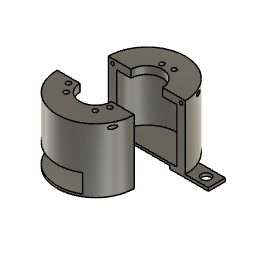
RotaryEncoderHolderCombined (Autodesk Fusion 360 design; units mm, degrees)
Autodesk Fusion 360 part; units mm, degrees
note: some values were not read from the file. Set by a fixed rule: which sketch regions a step uses.
sketch "Sketch1" plane through (0, 0, 0) normal (0, 0, 1) x (1, 0, 0)
  arc A0 (-25, 0) -> (25, 0) centre (0, 0) ccw
  line L0 (-25, 0) -> (25, 0)
  dimension "d3" = 50
  constraint coincident A0.centre origin
  constraint horizontal L0
  measures "d3" distance of A0.start A0.end
extrude "Extrude1" add sketch "Sketch1" along normal blind 41.5 makes body 1
sketch "Sketch2" plane through (0, 0, 41.5) normal (0, 0, 1) x (-1, 0, 0)
  arc A0 (25, 0) -> (-25, 0) centre (0, 0) ccw
  line L0 (-25, 0) -> (25, 0)
  circle A1 centre (0, 0) radius 19.5
  dimension "d6" = 39
  constraint coincident A0.centre A1.centre
  measures "d6" diameter of A1
extrude "Extrude2" cut sketch "Sketch2" against normal blind 35 from surface at -5 contours L0 A1 picked at (5.8563, 2.8202) bodies 1
sketch "Sketch5" plane through (0, 0, 41.5) normal (0, 0, 1) x (-1, 0, 0)
  arc A0 (25, 0) -> (-25, 0) centre (0, 0) ccw
  line L0 (-25, 0) -> (25, 0)
  circle A1 centre (0, 0) radius 10.25
  dimension "d10" = 20.5
  constraint coincident A0.centre A1.centre
  measures "d10" diameter of A1
extrude "Extrude3" cut sketch "Sketch5" against normal blind 5 contours L0 A1 picked at (0.2553, 3.4071) bodies 1
ref_plane "WorkPlane1" through (0, 0, 0) normal (0, 1, 0) x (0, 0, 1)
sketch "Sketch8" plane through (0, 0, 0) normal (0, 1, 0) x (-1, 0, 0)
  line L0 (-10.25, 36.5) -> (-10.25, 41.5)
  line L1 (-10.25, 41.5) -> (-25, 41.5)
  line L2 (-25, 41.5) -> (-25, 0)
  line L3 (-25, 0) -> (25, 0)
  line L4 (25, 0) -> (25, 41.5)
  line L5 (25, 41.5) -> (10.25, 41.5)
  line L6 (10.25, 41.5) -> (10.25, 36.5)
  line L7 (10.25, 36.5) -> (19.5, 36.5)
  line L8 (19.5, 36.5) -> (19.5, 1.5)
  line L9 (19.5, 1.5) -> (-19.5, 1.5)
  line L10 (-19.5, 1.5) -> (-19.5, 36.5)
  line L11 (-19.5, 36.5) -> (-10.25, 36.5)
  circle A0 centre (22.25, 38.75) radius 1.1
  line L12 (0, 46.5) -> (0, -12.5) construction
  line L13 (-30, 19) -> (33, 19) construction
  circle A1 centre (-22.25, 38.75) radius 1.1
  dimension "d40" = 2.2
  dimension "d41" = 2.75
  dimension "d42" = 2.75
  dimension "d43" = 22.5
  dimension "d44" = 22.25
  constraint perpendicular L3 L12
  constraint horizontal L13
  constraint symmetric A0 L12 A1
  measures "d40" diameter of A0
  measures "d41" distance of L4 A0.centre
  measures "d42" distance of L5 A0.centre
  measures "d43" distance of L1 L13
  measures "d44" distance of A0.centre L12
extrude "Extrude5" cut sketch "Sketch8" against normal blind 14 contours A0 | A1 bodies 1
mirror "Mirror1" about plane through (0, 0, 0) normal (0, 1, 0) of bodies 1 makes body 2
sketch "Sketch6" plane through (0, 0, 41.5) normal (0, 0, 1) x (-1, 0, 0)
  arc A0 (10.25, 0) -> (-10.25, 0) centre (0, 0) ccw
  line L0 (10.25, 0) -> (25, 0)
  arc A1 (25, 0) -> (-25, 0) centre (0, 0) ccw
  line L1 (-25, 0) -> (-10.25, 0)
  circle A2 centre (-12.968, 3.7525) radius 1.5
  circle A3 centre (-10.1336, 10.3711) radius 1.5
  circle A4 centre (14.0483, 3.5909) radius 1.5
  circle A5 centre (9.7334, 9.3547) radius 1.5
  dimension "d16" = 13.5
  dimension "d17" = 14.5
  dimension "d18" = 3
  dimension "d19" = 3
  dimension "d20" = 7.2
  dimension "d22" = 3
  dimension "d23" = 3
  dimension "d24" = 14.5
  dimension "d25" = 13.5
  dimension "d26" = 7.2
  dimension "d28" = 19.893
  dimension "d37" = 3.7525
  measures "d16" distance of A0.centre A2.centre
  measures "d17" distance of A0.centre A3.centre
  measures "d18" diameter of A2
  measures "d19" diameter of A3
  measures "d20" distance of A2.centre A3.centre
  measures "d22" diameter of A4
  measures "d23" diameter of A5
  measures "d24" distance of A0.centre A4.centre
  measures "d25" distance of A0.centre A5.centre
  measures "d26" distance of A4.centre A5.centre
  measures "d28" distance of A3.centre A5.centre
  measures "d37" distance of L1 A2.centre
ref_plane "WorkPlane2" through (0, -12.5, 41.5) normal (0, 0, 1) x (-1, 0, 0)
sketch "Sketch7" plane through (0, -11.5, 41.5) normal (0, 0, 1) x (1, 0, 0)
  circle A0 centre (-3.2352, 24.6066) radius 1.5
  circle A1 centre (3.9139, 25.4618) radius 1.5
  point P0 (0, 11.5)
  point P1 (-14.0483, 7.9091)
  dimension "d30" = 3
  dimension "d31" = 3
  dimension "d32" = 13.5
  dimension "d33" = 14.5
  dimension "d35" = 7.2
  dimension "d36" = 19.893
  measures "d30" diameter of A0
  measures "d31" diameter of A1
  measures "d32" distance of A0.centre P0
  measures "d33" distance of A1.centre P0
  measures "d35" distance of A0.centre A1.centre
  measures "d36" distance of A0.centre P1
extrude "Extrude4" cut sketch "Sketch6" sketch "Sketch7" against normal blind 5 contours A2 | A3 | A4 | A5 of sketch 2 bodies 1 2
sketch "Sketch9" plane through (0, 0, 0) normal (0, 0, -1) x (1, 0, 0)
  arc A0 (25, 0) -> (-25, 0) centre (0, 0) ccw
  line L0 (-25, 0) -> (25, 0)
  arc A1 (12.9192, 21.4032) -> (-25, 0) centre (0, 0) ccw
  line L1 (12.9192, 21.4032) -> (0, 0)
  constraint coincident A0.end L0.start
  constraint coincident A0.centre A1.centre
extrude "Extrude6" cut sketch "Sketch9" against normal blind 12 from surface at -1.5 contours A0 L0 A1 L1 bodies 1
sketch "Sketch10" plane through (0, 0, 0) normal (0, 0, -1) x (1, 0, 0)
  arc A0 (-25, 0) -> (25, 0) centre (0, 0) ccw
  line L0 (25, 0) -> (-25, 0)
  line L1 (-14.875, 0) -> (-40, 0)
  line L2 (-40, 0) -> (-40, -11)
  line L3 (-40, -11) -> (-14.875, -11)
  line L4 (-14.875, -11) -> (-14.875, 0)
  line L5 (-10.25, 0) -> (-19.5, 0)
  circle A1 centre (-33, -5.5) radius 3.1
  line L6 (0, 0) -> (0, -9) construction
  line L7 (14.875, -11) -> (14.875, 0)
  line L8 (40, -11) -> (14.875, -11)
  line L9 (14.875, 0) -> (40, 0)
  line L10 (40, 0) -> (40, -11)
  circle A2 centre (33, -5.5) radius 3.1
  dimension "d50" = 15
  dimension "d51" = 11
  dimension "d52" = 6.2
  dimension "d61" = 5.5
  dimension "d62" = 7
  constraint horizontal L1
  constraint vertical L2
  constraint horizontal L3
  constraint vertical L4
  constraint midpoint L1.start L5
  constraint coincident A0.centre L6.start
  constraint perpendicular L0 L6
  constraint symmetric L1.start L6 L7.end
  constraint symmetric L1.end L6 L9.end
  constraint symmetric L2.end L6 L8.start
  constraint symmetric L3.end L6 L7.start
  constraint symmetric A1 L6 A2
  measures "d50" distance of A0.start L1.end
  measures "d51" distance of L1.end L2.end
  measures "d52" diameter of A1
  measures "d61" distance of L1 A1.centre
  measures "d62" distance of L2 A1.centre
extrude "Extrude9" add sketch "Sketch10" along normal blind 2 contours A0 L0 L1 L3 L4 L5 | A0 L1 L2 L3 | A0 L0 L7 L8 L9 | A0 L8 L9 L10 bodies 2
move_body "Move3" bodies 2 to x (1, 0, 0) y (0, 1, 0) z (0, 0, 1) at (8.7347, 24.4851, 0)
